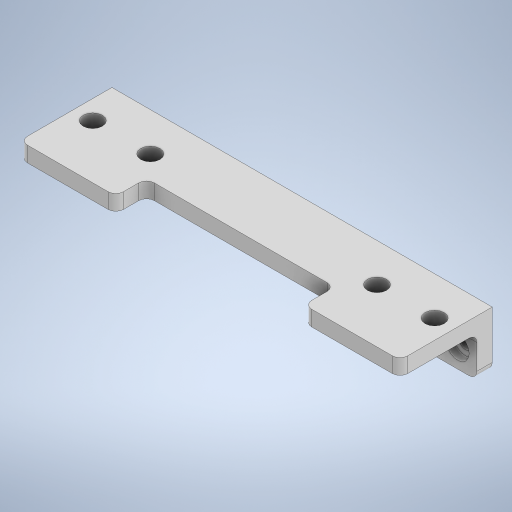
# Autodesk Inventor part: BP_L-Ver2
Saved by Autodesk Inventor 2024.3 (Build 283343000, 343)
## iProperties
Created: 2025-12-24
Part Number: BP_L-Ver2
Material: 一般
Document SubType Name: Modeling
Designer: 佐藤智貴
Density: 1 g/cm^3
Appearance: 既定
Author: 佐藤智貴
Autodesk Inventor part; units mm, degrees
ref_plane "YZ Plane" through (0, 0, 0) normal (1, 0, 0) x (0, 1, 0)
ref_plane "XZ Plane" through (0, 0, 0) normal (0, 1, 0) x (-1, 0, 0)
ref_plane "XY Plane" through (0, 0, 0) normal (0, 0, 1) x (1, 0, 0)
sketch "スケッチ1" plane through (0, 0, 0) normal (0, 0, 1) x (1, 0, 0)
  line L0 (0, 0) -> (25, 0)
  line L1 (25, 0) -> (25, 14.5)
  line L2 (25, 14.5) -> (0, 14.5)
  line L3 (0, 14.5) -> (0, 0)
  circle A0 centre (5, 5) radius 1.6
  circle A1 centre (20, 5) radius 1.6
  dimension "d0" = 3.2
  dimension "d1" = 3.2
  dimension "d2" = 15
  dimension "d3" = 5
  dimension "d4" = 5
  dimension "d5" = 9.5
  dimension "d6" = 14.5
  dimension "d7" = 9.5
  constraints: 8 end point, 2 centre point, 2 parallel, 1 horizontal, 1 perpendicular
  measures "d0" diameter of A0
  measures "d1" diameter of A1
  measures "d2" distance of A1.centre A0.centre
  measures "d3" distance from line of L3 A0.centre
  measures "d4" distance from line of L1 A1.centre
  measures "d5" distance from line of L2 A0.centre
  measures "d6" distance of L0.end L1.end
  measures "d7" distance from line of L2 A1.centre
extrude "押し出し1" add sketch "スケッチ1" along normal blind 4
sketch "スケッチ2" plane through (0, 0, 4) normal (0, 0, 1) x (1, 0, 0)
  line L0 (25, 14.5) -> (0, 14.5) projected
  line L1 (25, 0) -> (25, 14.5) projected
  line L2 (0, 14.5) -> (25, 14.5)
  line L3 (25, 14.5) -> (25, 10.5)
  line L4 (25, 10.5) -> (0, 10.5)
  line L5 (0, 10.5) -> (0, 14.5)
  point P0 (0, 0)
  dimension "d10" = 4
  constraints: 8 end point, 2 parallel, 1 horizontal, 1 perpendicular, 1 point on line
  measures "d10" distance between parallel lines of L0 L4
extrude "押し出し2" add sketch "スケッチ2" along normal blind 20
sketch "スケッチ3" plane through (0, 10.5, 4) normal (0, -1, 0) x (1, 0, 0)
  line L0 (0, 0) -> (0, 20) projected
  line L1 (0, 0) -> (25, 0) projected
  point P0 (0, -4)
  point P1 (5, 6)
  point P2 (20, 6)
  dimension "d13" = 15
  dimension "d14" = 5
  dimension "d15" = 6
  dimension "d16" = 6
  measures "d13" distance of point (20, 6) point (5, 6)
  measures "d14" distance from line of L0 point (5, 6)
  measures "d15" distance from line of L1 point (5, 6)
  measures "d16" distance from line of L1 point (20, 6)
hole "穴1" at (5, 10.5, 10) at (20, 10.5, 10) direction (0, 1, 0) diameter 5 end through all
sketch "スケッチ4" plane through (25, 0, 0) normal (1, 0, 0) x (0, 0, -1)
  line L0 (0, 0) -> (0, 14.5) projected
  line L1 (0, 14.5) -> (-24, 14.5) projected
  line L2 (-24, 10.5) -> (-24, 14.5) projected
  line L3 (-4, 10.5) -> (-24, 10.5) projected
  line L4 (-4, 0) -> (-4, 10.5) projected
  line L5 (0, 0) -> (-4, 0) projected
extrude "押し出し3" add sketch "スケッチ4" along normal blind 74
sketch "スケッチ5" plane through (0, 0, 4) normal (0, 0, 1) x (1, 0, 0)
  circle A0 centre (79, 5) radius 1.6
  circle A1 centre (94, 5) radius 1.6
  line L0 (0, 14.5) -> (99, 14.5) projected
  circle A2 centre (5, 5) radius 1.6 projected
  point P0 (0, 0)
  dimension "d26" = 3.2
  dimension "d27" = 3.2
  dimension "d28" = 15
  dimension "d29" = 9.5
  dimension "d30" = 9.5
  dimension "d31" = 89
  constraints: 2 centre point
  measures "d26" diameter of A1
  measures "d27" diameter of A0
  measures "d28" distance of A1.centre A0.centre
  measures "d29" distance from line of L0 A1.centre
  measures "d30" distance from line of L0 A0.centre
  measures "d31" distance of A2.centre A1.centre
extrude "押し出し4" cut sketch "スケッチ5" against normal blind 79 contours A0 | A1
sketch "スケッチ6" plane through (0, 10.5, 4) normal (0, -1, 0) x (1, 0, 0)
  line L0 (0, 20) -> (99, 20) projected
  line L1 (0, -4) -> (99, -4) projected
  line L2 (0, 20) -> (25, 20)
  line L3 (25, 20) -> (25, -4)
  line L4 (25, -4) -> (0, -4)
  line L5 (0, -4) -> (0, 20)
  line L6 (99, 20) -> (99, 0) projected
  line L7 (99, 20) -> (74, 20)
  line L8 (74, 20) -> (74, -4)
  line L9 (74, -4) -> (99, -4)
  line L10 (99, -4) -> (99, 20)
  line L11 (25, 20) -> (74, 20)
  line L12 (74, 20) -> (74, 12)
  line L13 (74, 12) -> (25, 12)
  line L14 (25, 12) -> (25, 20)
  circle A0 centre (79, 6) radius 2.5
  circle A1 centre (94, 6) radius 2.5
  line L15 (0, 0) -> (99, 0) projected
  circle A2 centre (20, 6) radius 2.5 projected
  point P0 (25, 20)
  dimension "d34" = 25
  dimension "d35" = 25
  dimension "d36" = 8
  dimension "d37" = 6
  dimension "d38" = 5
  dimension "d39" = 5
  dimension "d40" = 15
  dimension "d41" = 5
  dimension "d42" = 6
  dimension "d43" = 6
  constraints: 24 end point, 6 parallel, 3 horizontal, 3 perpendicular, 3 point on line, 2 centre point
  measures "d34" distance between parallel lines of L5 L3
  measures "d35" distance between parallel lines of L6 L8
  measures "d36" distance between parallel lines of L13 L0
  measures "d37" distance from line of L15 A2.centre
  measures "d38" diameter of A0
  measures "d39" diameter of A1
  measures "d40" distance of A1.centre A0.centre
  measures "d41" distance from line of L8 A0.centre
  measures "d42" distance from line of L15 A1.centre
  measures "d43" distance from line of L15 A0.centre
extrude "押し出し5" cut sketch "スケッチ6" against normal blind 74 contours L0 L8 L13 L3 | A0 | A1
fillet "フィレット1" radius 2 8 edges at (0, 12.5, 24) (25, 12.5, 24) (25, 12.5, 16) (74, 12.5, 24) (99, 12.5, 24) (74, 12.5, 16) (0, 0, 2) (99, 0, 2)
sketch "スケッチ8" plane through (0, 0, 4) normal (0, 0, 1) x (1, 0, 0)
  line L0 (27, 10.5) -> (27, 14.5) projected
  line L1 (27, 10.5) -> (32, 10.5)
  line L2 (32, 10.5) -> (32, 0)
  line L3 (32, 0) -> (27, 0)
  line L4 (27, 0) -> (27, 10.5)
  line L5 (72, 14.5) -> (72, 10.5) projected
  line L6 (72, 10.5) -> (67, 10.5)
  line L7 (67, 10.5) -> (67, 0)
  line L8 (67, 0) -> (72, 0)
  line L9 (72, 0) -> (72, 10.5)
  point P0 (0, 0)
  dimension "d47" = 10.5
  dimension "d48" = 5
  dimension "d49" = 5
  constraints: 16 end point, 4 parallel, 2 horizontal, 2 perpendicular, 1 point on line
  measures "d47" distance of L1.end L2.end
  measures "d48" distance between parallel lines of L4 L2
  measures "d49" distance between parallel lines of L9 L7
extrude "押し出し6" add sketch "スケッチ8" along normal blind 12
sketch "スケッチ9" plane through (72, 0, 4) normal (1, 0, 0) x (0, 0, -1)
  line L0 (0, 10.5) -> (0, 0) projected
  line L1 (-12, 10.5) -> (0, 10.5) projected
  line L2 (-12, 0) -> (-12, 10.5) projected
  line L3 (0, 0) -> (-12, 0) projected
  line L4 (-12, 14.5) -> (-12, 10.5) projected
  line L5 (0, 0) -> (-12, 10.5)
  point P0 (4, 0)
  constraints: 2 end point
extrude "押し出し7" cut sketch "スケッチ9" against normal through all contours L3 L2 L5
fillet "フィレット2" radius 2 3 edges at (13.5, 10.5, 4) (49.5, 10.5, 4) (85.5, 10.5, 4)
sketch "スケッチ10" plane through (0, 0, 4) normal (0, 0, 1) x (1, 0, 0)
  line L0 (0, 8.5) -> (27, 8.5) projected
  line L1 (0, 8.5) -> (0, 2) projected
  arc A0 (0, 2) -> (2, 0) centre (2, 2) ccw projected
  line L2 (2, 0) -> (27, 0) projected
  line L3 (27, 0) -> (27, 8.5) projected
  circle A1 centre (20, 5) radius 1.6 projected
  circle A2 centre (5, 5) radius 1.6 projected
  circle A3 centre (94, 5) radius 1.6 projected
  circle A4 centre (79, 5) radius 1.6 projected
  line L4 (72, 8.5) -> (99, 8.5) projected
  line L5 (72, 8.5) -> (72, 0) projected
  line L6 (72, 0) -> (97, 0) projected
  arc A5 (97, 0) -> (99, 2) centre (97, 2) ccw projected
  line L7 (99, 8.5) -> (99, 2) projected
  circle A6 centre (5, 5) radius 1.6 projected
  circle A7 centre (5, 5) radius 3
  circle A8 centre (20, 5) radius 3
  circle A9 centre (79, 5) radius 3
  circle A10 centre (94, 5) radius 3
  point P0 (0, 0)
  dimension "d55" = 6
  dimension "d56" = 6
  dimension "d57" = 6
  dimension "d58" = 6
  constraints: 4 centre point
  measures "d55" diameter of A9
  measures "d56" diameter of A10
  measures "d57" diameter of A7
  measures "d58" diameter of A8
extrude "押し出し8" cut sketch "スケッチ10" against normal blind 2 contours A1 | A2 | A4 | A7 | A8 | A9 | A10
equation "\"d1\" = d0"
equation "\"d4\" = d3"
equation "\"d16\" = d15"
equation "\"d27\" = d26"
equation "\"d30\" = d29"
equation "\"d35\" = d34"
equation "\"d39\" = d38"
equation "\"d43\" = d42"
equation "\"d49\" = d48"
equation "\"d56\" = d55"
equation "\"d58\" = d57"
